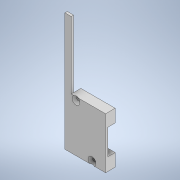
# Autodesk Inventor part: servoholder
Saved by Autodesk Inventor 2022 (Build 260153000, 153)
## iProperties
Created: 2021-01-11
Part Number: servoholder
Material: Generic
Document SubType Name: Modeling
Designer: papa
Density: 1 g/cm^3
Appearance: Default
Author: papa
Autodesk Inventor part; units mm, degrees
ref_plane "YZ Plane" through (0, 0, 0) normal (1, 0, 0) x (0, 1, 0)
ref_plane "XZ Plane" through (0, 0, 0) normal (0, 1, 0) x (-1, 0, 0)
ref_plane "XY Plane" through (0, 0, 0) normal (0, 0, 1) x (1, 0, 0)
sketch "Sketch1" plane through (0, 0, 0) normal (0, 0, 1) x (1, 0, 0)
  line L0 (5.5, 34.5) -> (27, 34.5)
  line L1 (1.5, 2.5) -> (27, 2.5)
  line L2 (27, 2.5) -> (27, 34.5)
  line L3 (27, 34.5) -> (5.5, 34.5)
  line L4 (1.5, 35.5) -> (1.5, 2.5)
  line L5 (1.5, 76.5) -> (5.5, 76.5)
  line L6 (1.5, 2.5) -> (5.5, 2.5)
  line L7 (5.5, 34.5) -> (5.5, 76.5)
  line L8 (5.5, 76.5) -> (1.5, 76.5)
  line L9 (1.5, 76.5) -> (1.5, 2.5)
  point P0 (0, 0)
  dimension "d0" = 32
  dimension "d2" = 21.5
  dimension "d3" = 42
  dimension "d17" = 4
  constraints: 20 end point, 4 parallel, 2 horizontal, 2 perpendicular
  measures "d0" distance between parallel lines of L1 L0
  measures "d2" distance of L0.start L0.end
  measures "d3" distance of L0.start L5.end
  measures "d17" distance between parallel lines of L7 L9
extrude "Extrusion1" add sketch "Sketch1" along normal blind 1.5
sketch "Sketch2" plane through (0, 0, 0) normal (0, 0, -1) x (-1, 0, 0)
  line L0 (-27, 2.5) -> (-27, 34.5) projected
  line L1 (-27, 34.5) -> (-5.5, 34.5)
  line L2 (-5.5, 34.5) -> (-5.5, 26.5)
  line L3 (-5.5, 26.5) -> (-27, 26.5)
  line L4 (-27, 26.5) -> (-27, 34.5)
  line L5 (-1.5, 2.5) -> (-27, 2.5) projected
  line L6 (-27, 2.5) -> (-5.5, 2.5)
  line L7 (-5.5, 2.5) -> (-5.5, 10.5)
  line L8 (-5.5, 10.5) -> (-27, 10.5)
  line L9 (-27, 10.5) -> (-27, 2.5)
  point P0 (0, 0)
  point P1 (-27, 10.5)
  point P2 (-27, 26.5)
  dimension "d6" = 16
  constraints: 16 end point, 4 parallel, 2 horizontal, 2 perpendicular, 1 collinear, 1 point on line
  measures "d6" distance between parallel lines of L8 L3
extrude "Extrusion2" add sketch "Sketch2" along normal blind 4.5
sketch "Sketch3" plane through (0, 0, 1.5) normal (0, 0, 1) x (1, 0, 0)
  circle A0 centre (8.5, 32.5) radius 1
  circle A1 centre (18.5, 4.5) radius 1
  line L0 (27, 2.5) -> (27, 34.5) projected
  line L1 (1.5, 2.5) -> (27, 2.5) projected
  line L2 (27, 34.5) -> (5.5, 34.5) projected
  point P0 (0, 0)
  dimension "d9" = 2
  dimension "d10" = 2
  dimension "d11" = 18.5
  dimension "d12" = 8.5
  dimension "d13" = 2
  dimension "d14" = 2
  constraints: 2 centre point
  measures "d9" diameter of A0
  measures "d10" diameter of A1
  measures "d11" distance from line of L0 A0.centre
  measures "d12" distance from line of L0 A1.centre
  measures "d13" distance from line of L1 A1.centre
  measures "d14" distance from line of L2 A0.centre
extrude "Extrusion3" cut sketch "Sketch3" against normal through all
chamfer "Chamfer1" distance 1.5 angle 45 2 edges at (7.5, 32.5, 1.5) (17.5, 4.5, 1.5)
body "Solid1"
